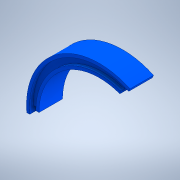
# Autodesk Inventor part: buttons_button_cap
Saved by Autodesk Inventor 2020 (Build 240168000, 168)
## iProperties
Created: 2019-11-16
Part Number: buttons_button_cap
Material: Generic
Document SubType Name: Modeling
Designer: suchanek
Density: 1 g/cm^3
Appearance: Default
Author: suchanek
Autodesk Inventor part; units mm, degrees
ref_plane "YZ Plane" through (0, 0, 0) normal (1, 0, 0) x (0, 1, 0)
ref_plane "XZ Plane" through (0, 0, 0) normal (0, 1, 0) x (-1, 0, 0)
ref_plane "XY Plane" through (0, 0, 0) normal (0, 0, 1) x (1, 0, 0)
sketch "Sketch1" plane through (0, 0, 0) normal (0, 1, 0) x (-1, 0, 0)
  line L0 (0, 0) -> (0, 10.6213)
  line L1 (19.2, 0) -> (20.2, 0)
  line L2 (20.2, 0) -> (20.2, 7.5)
  line L3 (20.2, 7.5) -> (19.2, 7.5)
  line L4 (19.2, 7.5) -> (19.2, 0)
  line L5 (20.2, 6.4) -> (22.2, 6.4)
  line L6 (22.2, 6.4) -> (22.2, 1.1)
  line L7 (22.2, 1.1) -> (20.2, 1.1)
  line L8 (20.2, 1.1) -> (20.2, 6.4)
  line L9 (22.2, 7.5) -> (23.2, 7.5)
  line L10 (23.2, 7.5) -> (23.2, 0)
  line L11 (23.2, 0) -> (22.2, 0)
  line L12 (22.2, 0) -> (22.2, 7.5)
  point P0 (22.2, 1.1)
  point P1 (22.2, 1.1)
  dimension "d0" = 1
  dimension "d1" = 7.5
  dimension "d2" = 2
  dimension "d3" = 1
  dimension "d4" = 1.1
  dimension "d5" = 1.1
  dimension "d6" = 20.2
  constraints: 26 end point, 6 parallel, 5 point on line, 3 horizontal, 3 perpendicular, 1 vertical
  measures "d0" distance of L3.end L2.end
  measures "d1" distance of L2.end L1.end
  measures "d2" distance of L6.end L7.end
  measures "d3" distance of L10.end L11.end
  measures "d4" distance between parallel lines of L1 L7
  measures "d5" distance between parallel lines of L3 L5
  measures "d6" distance between parallel lines of L2 L0
revolve "Revolution1" add sketch "Sketch1" angle 110 about axis through (0, 0, 0) along (0, 0, -1)
revolve "Revolution2" add sketch "Sketch1" angle 5 about axis through (0, 0, 0) along (0, 0, 1) and the other way 115 contours L6 L12 L9 L10 L11
body "Solid1"
